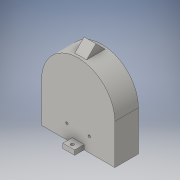
# Autodesk Inventor part: Tail1
Saved by Autodesk Inventor 2016 (Build 200138000, 138)
## iProperties
Created: 2017-03-09
Part Number: Tail1
Material: Generic
Document SubType Name: Modeling
Designer: Owner
Density: 1 g/cm^3
Appearance: Default
Author: Owner
Autodesk Inventor part; units mm, degrees
ref_plane "YZ Plane" through (0, 0, 0) normal (1, 0, 0) x (0, 1, 0)
ref_plane "XZ Plane" through (0, 0, 0) normal (0, 1, 0) x (-1, 0, 0)
sketch "Sketch1" plane through (0, 0, 0) normal (0, 0, 1) x (1, 0, 0)
  line L0 (0, 38.1) -> (5, 38.1) projected
  line L1 (0, 0) -> (0, 38.1) projected
  line L2 (0, 0) -> (86.2, 0) projected
  line L3 (86.2, 0) -> (86.2, 38.1) projected
  line L4 (81.2, 38.1) -> (86.2, 38.1) projected
  arc A0 (81.2, 38.1) -> (5, 38.1) centre (43.1, 38.1) ccw projected
  arc A1 (86.2, 38.1) -> (0, 38.1) centre (43.1, 38.1) ccw projected
  line L5 (86.2, -5) -> (0, -5) projected
  circle A2 centre (43.1, 38.1) radius 39.37
  line L6 (3.73, 38.1) -> (83.74, 38.1)
  line L7 (83.74, -5) -> (3.73, -5)
  line L8 (3.73, -5) -> (3.73, 38.1)
  line L9 (81.2, 38.1) -> (3.73, 38.1)
  line L10 (3.73, 38.1) -> (3.73, -5)
  line L11 (3.73, -5) -> (81.2, -5)
  line L12 (82.47, 38.1) -> (3.73, 38.1)
  line L13 (3.73, 38.1) -> (3.73, -5)
  line L14 (3.73, -5) -> (82.47, -5)
  line L15 (82.47, -5) -> (82.47, 38.1)
  dimension "d3" = 78.74
  constraints: 20 end point, 4 parallel, 3 horizontal, 3 point on line, 2 perpendicular, 2 point on circle, 1 centre point, 1 coincident
  measures "d3" diameter of A2
extrude "Extrusion1" add sketch "Sketch1" along normal blind 25.4 contours A2 L4 A0 L0 | L0 L6 L4 A2 L2 | A2 L2 L8 | A0 L6 | L15 L2 A2 | A2 L2 L15 L5 L8 | L2 A2
sketch "Sketch2" plane through (0, 0, 0) normal (0, 0, -1) x (-1, 0, 0)
  line L0 (-34.95, -5) -> (-47.65, -5) projected
  line L1 (-47.65, -5) -> (-47.65, 0) projected
  line L2 (-47.65, 0) -> (-34.95, 0) projected
  line L3 (-34.95, 0) -> (-34.95, -5) projected
  line L4 (-3.73, 38.1) -> (-3.73, -5) projected
  line L5 (-3.73, -5) -> (-82.47, -5) projected
  line L6 (-82.47, -5) -> (-3.73, -5)
  line L7 (-43.1, -5) -> (-43.1, 0)
  line L8 (-43.1, 0) -> (-43.1, 5.0038)
  line L9 (-43.1, 5.0038) -> (-36.75, 5.0038)
  line L10 (-36.75, 5.0038) -> (-49.45, 5.0038)
  line L11 (-49.45, 5.0038) -> (-36.75, 5.0038)
  line L12 (-36.75, 5.0038) -> (-36.75, 0)
  line L13 (-36.75, 0) -> (-49.45, 0)
  line L14 (-49.45, 0) -> (-49.45, 5.0038)
  point P0 (0, 0)
  dimension "d44" = 5.0038
  dimension "d45" = 6.35
  dimension "d46" = 12.7
  dimension "d63" = 12.7
  constraints: 18 end point, 4 point on line, 3 horizontal, 2 parallel, 2 perpendicular, 1 midpoint
  measures "d44" distance of L7.end L8.end
  measures "d45" distance of L8.end L9.end
  measures "d46" distance of L9.end L10.end
  measures "d63" distance between parallel lines of L12 L14
extrude "Extrusion2" add sketch "Sketch2" along normal blind 10.16 contours L8 L9 L12 L2 | L2 L13 L14 L10 L8
sketch "Sketch4" plane through (0, 0, 25.4) normal (0, 0, 1) x (1, 0, 0)
  line L0 (3.73, -5) -> (82.47, -5) projected
  line L1 (43.1, -5) -> (49.45, -5)
  line L2 (49.45, -5) -> (36.75, -5)
  line L3 (36.75, -5) -> (49.45, -5)
  line L4 (49.45, -5) -> (49.45, 0)
  line L5 (49.45, 0) -> (36.75, 0)
  line L6 (36.75, 0) -> (36.75, -5)
  point P0 (0, 0)
  dimension "d56" = 6.35
  dimension "d57" = 12.7
  dimension "d62" = 12.7
  constraints: 12 end point, 2 parallel, 2 point on line, 1 horizontal, 1 midpoint, 1 perpendicular
  measures "d56" distance of L1.start L1.end
  measures "d57" distance of L1.end L2.end
  measures "d62" distance between parallel lines of L4 L6
extrude "Extrusion4" add sketch "Sketch4" along normal blind 10.16
ref_plane "Work Plane1" through (43.1, -5, 0) normal (-1, 0, 0) x (0, 0, 1)
sketch "Sketch9" plane through (43.1, -5, 0) normal (-1, 0, 0) x (0, 0, 1)
  line L0 (0, 82.47) -> (0, 43.1) projected
  line L1 (0, 82.47) -> (2.7051, 82.47)
  line L2 (0, 82.47) -> (25.4, 82.47) projected
  line L3 (2.7051, 82.47) -> (22.6949, 82.47)
  line L4 (22.6949, 82.47) -> (12.6873, 82.47)
  line L5 (12.6873, 82.47) -> (12.6873, 92.4776)
  line L6 (12.6873, 92.4776) -> (22.6949, 82.47)
  line L7 (12.6873, 92.4776) -> (2.7051, 82.47)
  point P0 (0, 5)
  dimension "d30" = 2.7051
  dimension "d31" = 19.9898
  dimension "d32" = 10.0076
  dimension "d33" = 10.0076
  constraints: 12 end point, 3 point on line, 1 perpendicular
  measures "d30" distance of L0.start L1.end
  measures "d31" distance of L1.end L3.end
  measures "d32" distance of L3.end L4.end
  measures "d33" distance of L4.end L5.end
extrude "Extrusion8" add sketch "Sketch9" along normal mid plane 12.7
sketch "Sketch11" plane through (36.75, 5.0038, 0) normal (0, 1, 0) x (1, 0, 0)
  line L0 (12.7, 10.16) -> (0, 10.16) projected
  line L1 (6.35, 10.16) -> (6.35, 6.35)
  circle A0 centre (6.35, 6.35) radius 2.2479
  point P0 (-36.75, 0)
  dimension "d47" = 3.81
  dimension "d48" = 4.4958
  constraints: 2 end point, 1 centre point, 1 coincident, 1 midpoint, 1 vertical
  measures "d47" distance of L1.start L1.end
  measures "d48" diameter of A0
extrude "Extrusion10" cut sketch "Sketch11" against normal blind 25.4
sketch "Sketch12" plane through (0, 0, 0) normal (0, 0, -1) x (-1, 0, 0)
  line L0 (-31.035, 12.5599) -> (-55.165, 12.5599) projected
  line L1 (-55.165, 8.4959) -> (-31.035, 8.4959) projected
  line L2 (-55.165, 12.5599) -> (-55.165, 8.4959)
  line L3 (-31.035, 12.5599) -> (-31.035, 8.4959)
  circle A0 centre (-55.165, 10.5279) radius 1.25
  circle A1 centre (-31.035, 10.5279) radius 1.25
  point P0 (0, 0)
  dimension "d51" = 2.5
  dimension "d52" = 2.5
  constraints: 4 end point, 2 centre point, 2 midpoint, 1 parallel, 1 vertical
  measures "d51" diameter of A0
  measures "d52" diameter of A1
extrude "Extrusion11" cut sketch "Sketch12" against normal blind 25.4 contours A1 L3 | L3 A1 | A0 L2 | L2 A0
sketch "Sketch13" plane through (36.75, 0, 25.4) normal (0, 1, 0) x (1, 0, 0)
  line L0 (0, -10.16) -> (12.7, -10.16) projected
  line L1 (6.35, -10.16) -> (6.35, -6.35)
  circle A0 centre (6.35, -6.35) radius 1.7526
  point P0 (-36.75, 25.4)
  dimension "d58" = 3.81
  dimension "d59" = 3.5052
  constraints: 2 end point, 1 centre point, 1 coincident, 1 midpoint, 1 vertical
  measures "d58" distance of L1.start L1.end
  measures "d59" diameter of A0
extrude "Extrusion12" cut sketch "Sketch13" against normal blind 25.4
body "Solid1"
